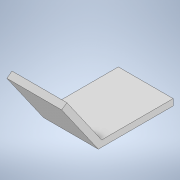
# Autodesk Inventor part: shooter bracket without motor
Saved by Autodesk Inventor 2021 (Build 250183000, 183)
## iProperties
Created: 2021-03-12
Part Number: shooter bracket without motor
Material: Generic
Document SubType Name: Modeling
Designer: deli
Density: 1 g/cm^3
Appearance: Default
Author: deli
Autodesk Inventor part; units mm, degrees
ref_plane "YZ Plane" through (0, 0, 0) normal (1, 0, 0) x (0, 1, 0)
ref_plane "XZ Plane" through (0, 0, 0) normal (0, 1, 0) x (-1, 0, 0)
ref_plane "XY Plane" through (0, 0, 0) normal (0, 0, 1) x (1, 0, 0)
sketch "Sketch1" plane through (0, 0, 0) normal (1, 0, 0) x (0, 1, 0)
  line L0 (104, 124.9907) -> (104, 66.293)
  line L1 (239.8243, 220.0959) -> (104, 124.9907)
  line L2 (227.1683, 205.1302) -> (109, 122.3878)
  line L3 (109, 122.3878) -> (109, 66.293)
  line L4 (144.9576, 153.6695) -> (147.8255, 149.5737)
  line L5 (109, 66.293) -> (104, 66.293)
  point P0 (0, 0)
  dimension "d2" = 58.6977
  dimension "d3" = 50
  constraints: 12 end point, 2 perpendicular, 2 point on line, 1 vertical, 1 other
  measures "d2" distance of L0.start L0.end
  measures "d3" distance from line of L0.start L4
extrude "Extrusion1" add sketch "Sketch1" along normal blind 43
body "Solid1"
